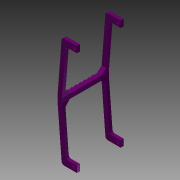
# Autodesk Inventor part: spacer
Saved by Autodesk Inventor 2015 (Build 190159000, 159)
## iProperties
Created: 2015-01-16
Part Number: spacer
Material: Generic
Document SubType Name: Modeling
Designer: Rafi Kurnia Putra
Density: 1 g/cm^3
Appearance: Smooth - Purple
Author: Rafi Kurnia Putra
Autodesk Inventor part; units mm, degrees
ref_plane "XZ Plane" through (0, 0, 0) normal (0, 1, 0) x (-1, 0, 0)
sketch "Sketch3" plane through (0, 0, 0) normal (0, 1, 0) x (-1, 0, 0)
  line L0 (17.0822, 51.9629) -> (21.0892, 2.5)
  line L1 (26.0892, 2.5) -> (21.5152, 58.9629)
  line L2 (4.3564, 54.5367) -> (14.274, 54.5367)
  arc A0 (21.5152, 58.9629) -> (18.6927, 61.5367) centre (18.7243, 58.7368) ccw
  line L3 (11.3604, 61.5367) -> (18.6927, 61.5367)
  circle A1 centre (7.8584, 58.0367) radius 1.75
  line L4 (11.3604, 61.5367) -> (7.8604, 61.5367)
  line L5 (4.3604, 61.5367) -> (11.3604, 61.5367)
  line L6 (4.3564, 54.5367) -> (4.3604, 61.5367)
  arc A2 (17.0822, 51.9629) -> (14.274, 54.5367) centre (14.2916, 51.737) ccw
  line L7 (26.0892, 2.5) -> (26.0892, 0)
  line L8 (26.0892, 2.5) -> (28.5892, 2.5) construction
  line L9 (21.0892, 2.5) -> (21.0892, 0)
  line L10 (26.0892, -2.5) -> (21.5112, -58.963)
  line L11 (17.0822, -51.9629) -> (21.0926, -2.5003)
  arc A3 (14.2916, -54.5367) -> (17.0822, -51.9629) centre (14.2916, -51.737) ccw
  line L12 (4.3564, -54.5367) -> (14.2916, -54.5367)
  arc A4 (18.6888, -61.5367) -> (21.5112, -58.963) centre (18.7203, -58.7369) ccw
  line L13 (11.3564, -61.5407) -> (18.6888, -61.5367)
  circle A5 centre (7.8584, -58.0367) radius 1.75
  line L14 (11.3564, -61.5407) -> (7.8564, -61.5387)
  line L15 (4.3564, -61.5367) -> (11.3564, -61.5407)
  line L16 (4.3564, -54.5367) -> (4.3564, -61.5367)
  line L17 (26.0892, -2.5) -> (26.0892, 0)
  line L18 (21.0892, -2.5) -> (21.0892, 0)
  line L19 (26.0892, -2.5) -> (26.0892, 2.5)
  line L20 (21.0892, -2.5) -> (21.0892, 2.5)
  line L21 (26.0892, -2.5) -> (26.0892, 2.5)
  line L22 (26.0892, 2.5) -> (21.5152, 58.9629)
  arc A6 (21.5152, 58.9629) -> (18.6927, 61.5367) centre (18.7243, 58.7368) ccw
  line L23 (4.3604, 61.5367) -> (18.6927, 61.5367)
  line L24 (4.3604, 61.5367) -> (4.3564, 54.5367)
  arc A7 (17.0822, 51.9629) -> (14.274, 54.5367) centre (14.2916, 51.737) ccw
  line L25 (17.0822, 51.9629) -> (21.0892, 2.5)
  line L26 (21.0892, -2.5) -> (17.0822, -51.9629)
  arc A8 (14.2916, -54.5367) -> (17.0822, -51.9629) centre (14.2916, -51.737) ccw
  line L27 (4.3564, -54.5367) -> (14.2916, -54.5367)
  line L28 (4.3564, -61.5367) -> (4.3564, -54.5367)
  line L29 (4.3564, -61.5367) -> (18.6888, -61.5367)
  arc A9 (18.6888, -61.5367) -> (21.5112, -58.963) centre (18.7203, -58.7369) ccw
  line L30 (21.5112, -58.963) -> (26.0892, -2.5)
  point P0 (0, 0)
  point P1 (16.8737, 54.5367)
  point P2 (16.8735, -54.5367)
  dimension "d0" = 7
  dimension "d1" = 3.5
  dimension "d2" = 7
  dimension "d8" = 3.5
  dimension "d9" = 3.5
  dimension "d13" = 9.9177
  dimension "d14" = 4.9837
  dimension "d15" = 8.2856
  dimension "d17" = 2.5
  dimension "d18" = 90
  dimension "d19" = 2.5
  dimension "d21" = 5
  dimension "d22" = 175.369
  dimension "d24" = 56.4629
  dimension "d25" = 49.4629
  dimension "d26" = 175.369
  dimension "d27" = 94.631
  dimension "d28" = 94.631
  dimension "d29" = 2.8
  dimension "d30" = 2.8
  dimension "d31" = 5
  constraints: 62 end point, 16 point on circle, 10 centre point, 9 collinear, 6 coincident, 5 tangent, 4 point on line, 3 perpendicular, 2 horizontal alignment, 2 parallel, 2 vertical, 1 horizontal
  measures "d0" distance of L2.start L5.start
  measures "d1" diameter of A1
  measures "d2" distance of L5.start L3.start
  measures "d8" distance from line of L5 A1.centre
  measures "d9" distance from line of L6 A1.centre
  measures "d13" distance of L2.start L2.end
  measures "d14" distance between parallel lines of L0 L1
  measures "d17" distance of L1.start L7.end
  measures "d18" angle of L7 L8
  measures "d19" distance of L9.start L9.end
  measures "d21" distance between parallel lines of L9 L7
  measures "d22" angle of L1 L7
  measures "d24" vertical distance of L1.start L1.end
  measures "d25" vertical distance of L0.start L0.end
  measures "d26" angle of L0 L9
  measures "d27" angle of L3 L1
  measures "d28" angle of L2 L0
  measures "d29" distance from line of A0.centre L1
  measures "d30" radius of A0
  measures "d31" distance of L1.start L10.start
extrude "Extrusion1" add sketch "Sketch3" along normal blind 3.5 contours A2 L2 L6 L5 L4 L3 A0 L1 L7 L17 L10 A4 L29 L15 L16 L12 A3 L26 L18 L9 L0
sketch "Sketch4" plane through (0, 3.5, 0) normal (0, 1, 0) x (1, 0, 0)
  line L0 (-26.0892, 2.5) -> (-21.0892, 2.5)
  line L1 (-21.0892, 2.5) -> (-21.0892, -2.5)
  line L2 (-21.0892, -2.5) -> (-26.0892, -2.5)
  line L3 (-26.0892, -2.5) -> (-26.0892, 2.5)
  point P0 (0, 0)
  dimension "d34" = 5
  dimension "d35" = 5
  constraints: 8 end point, 2 parallel, 1 horizontal, 1 perpendicular
  measures "d34" distance of L1.end L2.end
  measures "d35" distance of L0.end L1.end
extrude "Extrusion2" add sketch "Sketch4" along normal blind 22.75
fillet "Fillet1" radius 0.25 2 edges at (-26.0892, 14.875, 2.5) (-26.0892, 14.875, -2.5)
ref_plane "Work Plane2" through (-23.5891, 0, 0) normal (1, 0, 0) x (0, 1, 0)
sketch "Sketch6" plane through (-23.5891, 0, 0) normal (1, 0, 0) x (0, 1, 0)
  line L0 (3.5, -2.5) -> (8.5, -2.5)
  line L1 (26.25, -2.5) -> (3.5, -2.5) projected
  line L2 (3.5, -2.5) -> (8.5, -2.5) construction
  line L3 (8.5, -2.5) -> (3.5, -7.5)
  line L4 (3.5, -2.5) -> (3.5, -51.9629) projected
  line L5 (3.5, -7.5) -> (3.5, -2.5)
  point P0 (0, 0)
  dimension "d41" = 5
  dimension "d42" = 0
  dimension "d43" = 45
  constraints: 8 end point, 3 collinear, 1 horizontal, 1 point on line
  measures "d41" distance of L0.start L0.end
  measures "d42" distance between parallel lines of L0 L2
  measures "d43" angle of L0 L3
extrude "Extrusion3" add sketch "Sketch6" along normal mid plane 7
sketch "Sketch7" plane through (-21.0892, 3.5, -2.5) normal (0, -1, 0) x (1, 0, 0.0000004)
  line L0 (1, 0) -> (0, 0)
  line L1 (1, -5) -> (1, 0)
  line L2 (1, 0) -> (1, -5) projected
  line L3 (1, 0) -> (0, 0)
  line L4 (0.405, -5) -> (1, -5)
  line L5 (0.405, -5) -> (1, -5) projected
  line L6 (0, 0) -> (0.405, -5)
  point P0 (21.0892, 2.5)
  constraints: 10 end point, 2 collinear, 1 horizontal, 1 perpendicular
extrude "Extrusion4" cut sketch "Sketch7" against normal through all
sketch "Sketch8" plane through (-27.0891, 3.5, -7.5) normal (0, -1, 0) x (1, 0, 0)
  line L0 (0, 0) -> (0, 5)
  line L1 (0, 5) -> (1, 5)
  line L2 (1, 5) -> (1.4054, 0)
  line L3 (5.5779, -51.463) -> (1, 5) projected
  line L4 (1.4054, 0) -> (0, 0)
  line L5 (0, 0) -> (1.4054, 0) projected
  point P0 (27.0891, 7.5)
  constraints: 8 end point, 2 collinear, 1 perpendicular, 1 vertical
extrude "Extrusion5" cut sketch "Sketch8" against normal through all
ref_plane "Work Plane3" through (0, 0, 0) normal (0, 0, 1) x (1, 0, 0)
mirror "Mirror1" about plane through (0, 0, 0) normal (0, 0, 1) of "Extrusion3", "Extrusion4", "Extrusion5"
mirror "Mirror2" about plane through (-23.5892, 26.25, 0) normal (0, 1, 0) of "Extrusion1", "Fillet1", "Extrusion2", "Extrusion3", "Extrusion4", "Extrusion5", "Mirror1"
sketch "Sketch9" plane through (-26.0892, 0, -2.5) normal (-1, 0, 0) x (0, 0, 1)
  line L0 (0, 0) -> (5, 0) projected
  line L1 (0, 52.5) -> (5, 52.5) projected
  line L2 (0.6761, 13.4145) -> (0.6761, 39.0855) construction
  line L3 (0.6761, 39.0855) -> (4.3239, 39.0855) construction
  line L4 (4.3239, 39.0855) -> (4.3239, 13.4145) construction
  line L5 (4.3239, 13.4145) -> (0.6761, 13.4145) construction
  line L6 (0.25, 26.25) -> (4.75, 26.25) projected
  line L7 (0, 3.5) -> (0.25, 3.5) projected
  line L8 (0, 0) -> (0, 3.5) projected
  line L9 (0, 0) -> (5, 0) projected
  line L10 (5, 0) -> (5, 3.5) projected
  line L11 (4.75, 3.5) -> (5, 3.5) projected
  line L12 (4.75, 49) -> (4.75, 3.5) projected
  line L13 (4.75, 49) -> (5, 49) projected
  line L14 (5, 52.5) -> (5, 49) projected
  line L15 (0, 52.5) -> (5, 52.5) projected
  line L16 (0, 52.5) -> (0, 49) projected
  line L17 (0, 49) -> (0.25, 49) projected
  line L18 (0.25, 3.5) -> (0.25, 49) projected
  line L19 (0, 52.5) -> (5, 0)
  line L20 (5, 0) -> (0, 0)
  line L21 (5, 52.5) -> (0, 0)
  line L22 (0.975, 11.1414) -> (0.975, 11.7022)
  spline S0 degree 2 poles (0.975, 11.7022) (0.975, 12.263) (1.0623, 12.6606) (1.4186, 12.9111) (1.807, 12.9111) knots 0 0 0 1 2 3 3 3
  spline S1 degree 2 poles (1.807, 12.9111) (2.1633, 12.9111) (2.4092, 12.7342) (2.4345, 12.4744) knots 0 0 0 1 2 2 2
  spline S2 degree 2 poles (2.4345, 12.4744) (2.492, 12.7089) (2.6873, 12.8721) (2.8505, 12.9111) (3.2206, 12.9111) knots 0 0 0 1 2 3 3 3
  line L23 (3.2206, 12.9111) -> (4.025, 12.9111)
  line L24 (4.025, 12.9111) -> (4.025, 12.1733)
  line L25 (4.025, 12.1733) -> (3.0114, 12.1733)
  spline S3 degree 2 poles (3.0114, 12.1733) (2.7678, 12.1733) (2.6505, 12.0975) (2.6505, 11.9343) knots 0 0 0 1 2 2 2
  line L26 (2.6505, 11.9343) -> (4.025, 11.9343)
  line L27 (4.025, 11.9343) -> (4.025, 11.1414)
  line L28 (4.025, 11.1414) -> (0.975, 11.1414)
  line L29 (1.4967, 11.9343) -> (2.1748, 11.9343)
  spline S4 degree 2 poles (2.1748, 11.9343) (2.1748, 12.0676) (2.1012, 12.1733) (1.899, 12.1733) knots 0 0 0 1 2 2 2
  line L30 (1.899, 12.1733) -> (1.7312, 12.1733)
  spline S5 degree 2 poles (1.7312, 12.1733) (1.5864, 12.1733) (1.4967, 12.0699) (1.4967, 11.9343) knots 0 0 0 1 2 2 2
  spline S6 degree 2 poles (2.7609, 17.7516) (3.2206, 17.7516) (3.6021, 17.7079) (3.9193, 17.4804) (4.0894, 17.092) (4.0894, 16.8345) knots 0 0 0 1 2 3 4 4 4
  spline S7 degree 2 poles (4.0894, 16.8345) (4.0894, 16.5886) (3.9285, 16.2002) (3.609, 15.9634) (3.232, 15.9175) (2.7609, 15.9175) knots 0 0 0 1 2 3 4 4 4
  line L31 (2.7609, 15.9175) -> (2.2391, 15.9175)
  spline S8 degree 2 poles (2.2391, 15.9175) (1.7794, 15.9175) (1.3979, 15.9611) (1.0807, 16.1887) (0.9106, 16.5771) (0.9106, 16.8345) knots 0 0 0 1 2 3 4 4 4
  spline S9 degree 2 poles (0.9106, 16.8345) (0.9106, 17.0805) (1.0715, 17.4689) (1.391, 17.7056) (1.768, 17.7516) (2.2391, 17.7516) knots 0 0 0 1 2 3 4 4 4
  line L32 (2.2391, 17.7516) -> (2.7609, 17.7516)
  spline S10 degree 2 poles (1.7588, 16.9586) (1.5473, 16.9586) (1.4278, 16.9127) (1.4278, 16.8391) knots 0 0 0 1 2 2 2
  spline S11 degree 2 poles (1.4278, 16.8391) (1.4278, 16.7771) (1.5243, 16.7104) (1.7588, 16.7104) knots 0 0 0 1 2 2 2
  line L33 (1.7588, 16.7104) -> (3.1815, 16.7104)
  spline S12 degree 2 poles (3.1815, 16.7104) (3.4481, 16.7104) (3.5722, 16.7541) (3.5722, 16.8322) knots 0 0 0 1 2 2 2
  spline S13 degree 2 poles (3.5722, 16.8322) (3.5722, 16.9127) (3.4297, 16.9586) (3.1608, 16.9586) knots 0 0 0 1 2 2 2
  line L34 (3.1608, 16.9586) -> (1.7588, 16.9586)
  line L35 (0.975, 20.7694) -> (0.975, 21.5601)
  spline S14 degree 2 poles (0.975, 21.5601) (0.975, 21.937) (1.0922, 22.3232) (1.4485, 22.5599) (1.8438, 22.5599) knots 0 0 0 1 2 3 3 3
  spline S15 degree 2 poles (1.8438, 22.5599) (2.1104, 22.5599) (2.3219, 22.3921) (2.377, 22.1439) knots 0 0 0 1 2 2 2
  spline S16 degree 2 poles (2.377, 22.1439) (2.4414, 22.4197) (2.7287, 22.6151) (3.0275, 22.6151) knots 0 0 0 1 2 2 2
  line L36 (3.0275, 22.6151) -> (3.3079, 22.6151)
  spline S17 degree 2 poles (3.3079, 22.6151) (3.6182, 22.6151) (3.9147, 22.4748) (4.025, 22.1646) (4.025, 21.6865) knots 0 0 0 1 2 3 3 3
  line L37 (4.025, 21.6865) -> (4.025, 20.7694)
  line L38 (4.025, 20.7694) -> (0.975, 20.7694)
  line L39 (2.6505, 21.5624) -> (3.5033, 21.5624)
  spline S18 degree 2 poles (3.5033, 21.5624) (3.4987, 21.7302) (3.4044, 21.8221) (3.2183, 21.8221) knots 0 0 0 1 2 2 2
  line L40 (3.2183, 21.8221) -> (2.9356, 21.8221)
  spline S19 degree 2 poles (2.9356, 21.8221) (2.7379, 21.8221) (2.6551, 21.7394) (2.6505, 21.5624) knots 0 0 0 1 2 2 2
  line L41 (1.4967, 21.5624) -> (2.1748, 21.5624)
  spline S20 degree 2 poles (2.1748, 21.5624) (2.1725, 21.6129) (2.1725, 21.6405) knots 0 0 0 1 1 1
  spline S21 degree 2 poles (2.1725, 21.6405) (2.1725, 21.7577) (2.0576, 21.8221) (1.7863, 21.8221) knots 0 0 0 1 2 2 2
  spline S22 degree 2 poles (1.7863, 21.8221) (1.6438, 21.8221) (1.5289, 21.7692) (1.499, 21.6842) (1.4967, 21.5624) knots 0 0 0 1 2 3 3 3
  line L42 (0.975, 27.4233) -> (3.0137, 27.4233)
  spline S23 degree 2 poles (3.0137, 27.4233) (3.3608, 27.4233) (3.6412, 27.3774) (3.9377, 27.1567) (4.0894, 26.7936) (4.0894, 26.5453) knots 0 0 0 1 2 3 4 4 4
  spline S24 degree 2 poles (4.0894, 26.5453) (4.0894, 26.2718) (3.9078, 25.8558) (3.6182, 25.6467) (3.2964, 25.6099) (2.7793, 25.6099) knots 0 0 0 1 2 3 4 4 4
  line L43 (2.7793, 25.6099) -> (0.975, 25.6099)
  line L44 (0.975, 25.6099) -> (0.975, 26.4028)
  line L45 (0.975, 26.4028) -> (3.2619, 26.4028)
  spline S25 degree 2 poles (3.2619, 26.4028) (3.4619, 26.4028) (3.5722, 26.4465) (3.5722, 26.5109) knots 0 0 0 1 2 2 2
  spline S26 degree 2 poles (3.5722, 26.5109) (3.5722, 26.5867) (3.4504, 26.6304) (3.2229, 26.6304) knots 0 0 0 1 2 2 2
  line L46 (3.2229, 26.6304) -> (0.975, 26.6304)
  line L47 (0.975, 26.6304) -> (0.975, 27.4233)
  line L48 (1.8967, 32.1328) -> (1.8967, 31.395)
  line L49 (1.8967, 31.395) -> (1.6714, 31.395)
  spline S27 degree 2 poles (1.6714, 31.395) (1.5151, 31.395) (1.4278, 31.3398) (1.4278, 31.2732) knots 0 0 0 1 2 2 2
  spline S28 degree 2 poles (1.4278, 31.2732) (1.4278, 31.2019) (1.545, 31.1284) (1.6622, 31.1284) knots 0 0 0 1 2 2 2
  spline S29 degree 2 poles (1.6622, 31.1284) (1.8139, 31.1284) (1.8921, 31.1698) knots 0 0 0 1 1 1
  spline S30 degree 2 poles (1.8921, 31.1698) (1.9702, 31.2111) (2.0782, 31.395) knots 0 0 0 1 1 1
  spline S31 degree 2 poles (2.0782, 31.395) (2.3931, 31.9236) (2.5954, 32.0615) knots 0 0 0 1 1 1
  spline S32 degree 2 poles (2.5954, 32.0615) (2.7976, 32.1995) (3.2458, 32.1995) knots 0 0 0 1 1 1
  spline S33 degree 2 poles (3.2458, 32.1995) (3.5722, 32.1995) (3.8802, 32.0478) (4.0894, 31.6088) (4.0894, 31.3192) knots 0 0 0 1 2 3 3 3
  spline S34 degree 2 poles (4.0894, 31.3192) (4.0894, 31.002) (3.848, 30.5515) (3.4757, 30.4113) (3.1332, 30.4113) knots 0 0 0 1 2 3 3 3
  line L50 (3.1332, 30.4113) -> (2.9333, 30.4113)
  line L51 (2.9333, 30.4113) -> (2.9333, 31.1491)
  line L52 (2.9333, 31.1491) -> (3.3033, 31.1491)
  spline S35 degree 2 poles (3.3033, 31.1491) (3.4734, 31.1491) (3.5722, 31.2111) (3.5722, 31.2893) knots 0 0 0 1 2 2 2
  spline S36 degree 2 poles (3.5722, 31.2893) (3.5722, 31.3697) (3.4481, 31.4456) (3.3263, 31.4456) knots 0 0 0 1 2 2 2
  spline S37 degree 2 poles (3.3263, 31.4456) (3.0574, 31.4456) (2.9746, 31.372) knots 0 0 0 1 1 1
  spline S38 degree 2 poles (2.9746, 31.372) (2.8919, 31.2962) (2.6965, 30.9997) knots 0 0 0 1 1 1
  spline S39 degree 2 poles (2.6965, 30.9997) (2.5011, 30.7055) (2.3242, 30.5124) (2.0116, 30.386) (1.768, 30.386) knots 0 0 0 1 2 3 3 3
  spline S40 degree 2 poles (1.768, 30.386) (1.4163, 30.386) (1.0922, 30.5653) (0.9106, 30.9652) (0.9106, 31.2479) knots 0 0 0 1 2 3 3 3
  spline S41 degree 2 poles (0.9106, 31.2479) (0.9106, 31.5559) (1.1106, 31.9926) (1.414, 32.1328) (1.7771, 32.1328) knots 0 0 0 1 2 3 3 3
  line L53 (1.7771, 32.1328) -> (1.8967, 32.1328)
  line L54 (0.975, 36.7664) -> (1.5864, 36.7664)
  line L55 (1.5864, 36.7664) -> (1.5864, 36.2952)
  line L56 (1.5864, 36.2952) -> (4.025, 36.2952)
  line L57 (4.025, 36.2952) -> (4.025, 35.5023)
  line L58 (4.025, 35.5023) -> (1.5864, 35.5023)
  line L59 (1.5864, 35.5023) -> (1.5864, 35.0334)
  line L60 (1.5864, 35.0334) -> (0.975, 35.0334)
  line L61 (0.975, 35.0334) -> (0.975, 36.7664)
  line L62 (0.975, 41.0392) -> (4.025, 41.4943)
  line L63 (4.025, 41.4943) -> (4.025, 40.6806)
  line L64 (4.025, 40.6806) -> (3.4757, 40.6392)
  line L65 (3.4757, 40.6392) -> (3.4757, 40.3565)
  line L66 (3.4757, 40.3565) -> (4.025, 40.3106)
  line L67 (4.025, 40.3106) -> (4.025, 39.4877)
  line L68 (4.025, 39.4877) -> (0.975, 39.89)
  line L69 (0.975, 39.89) -> (0.975, 41.0392)
  spline S42 degree 2 poles (2.9356, 40.6186) (2.4184, 40.5611) (1.6553, 40.499) knots 0 0 0 1 1 1
  spline S43 degree 2 poles (1.6553, 40.499) (2.531, 40.3795) (2.9356, 40.3473) knots 0 0 0 1 1 1
  line L70 (2.9356, 40.3473) -> (2.9356, 40.6186)
  point P0 (2.5, 0)
  point P1 (2.5, 26.25)
  point P2 (2.5, 26.25)
  point P3 (2.5, 26.25)
  point P4 (2.5, 26.25)
  dimension "d51" = 52.5
  dimension "d52" = 1.8238
  dimension "d53" = 12.8355
  constraints: 6 end point, 3 midpoint, 1 coincident, 1 collinear, 3 other
  measures "d51" distance between parallel lines of L0 L1
  measures "d52" distance from line of L2 point (2.5, 26.25)
  measures "d53" distance from line of L5 point (2.5, 26.25)
extrude "Extrusion6" add sketch "Sketch9" along normal blind 1.5 contours L28 L22 S0 L21 | L21 S0 S1 S2 L23 L19 L25 S3 L26 L28 | L19 L26 L27 L28 | S8 S9 L21 S10 S11 | L21 S11 L33 S12 L19 S7 L31 S8 | L19 L23 L24 L25 | L44 L45 L19 L6 | L6 L21 L43 L44 | S24 L43 L19 L6 | L6 L21 L45 S25 S26 L46 L42 S23 S24 | L19 L45 L21 | L19 L43 L21 | L21 S9 L32 S6 L19 S13 L34 S10 | L19 S12 S13 S6 S7 | L38 L35 S14 S15 L21 S21 S22 L41 | L21 L41 S20 S21 S15 S16 L19 S19 L39 L38 | L46 L47 L42 L19 | L19 L42 L21 L46 | S16 L36 S17 L37 L38 L19 L39 S18 L40 S19 | L62 L21 L64 L65 L66 L68 L19 | L19 L68 L69 L62 | L62 L63 L64 L21 | L51 L52 L21 | L21 L52 S35 S36 S37 S32 S33 S34 L50 L51 | S39 S40 S41 L53 L48 L49 S27 S28 S29 S30 L19 | L19 S30 S31 S32 L21 S37 S38 S39 | L54 L55 L56 L21 L58 L19 | L19 L58 L59 L60 L61 L54 | L21 L66 L67 L68 | L56 L57 L58 L21
body "Solid1"
